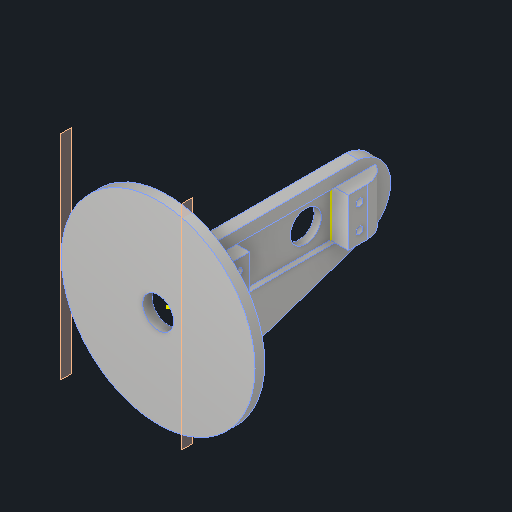
# Autodesk Inventor part: wrist
Saved by Autodesk Inventor 2023.4 (Build 274418000, 418)
## iProperties
Created: 2020-06-03
Part Number: wrist
Material: Aluminum 6061
Document SubType Name: Modeling
Designer: lenovo
Density: 2.7 g/cm^3
Appearance: Aluminum - Flat
Author: lenovo
Autodesk Inventor part; units mm, degrees
ref_plane "XZ Plane" through (0, 0, 0) normal (0, 1, 0) x (-1, 0, 0)
ref_plane "XY Plane" through (0, 0, 0) normal (0, 0, 1) x (1, 0, 0)
sketch "Sketch1" plane through (0, 0, 0) normal (0, 0, 1) x (1, 0, 0)
  circle A0 centre (0, 0) radius 40
  dimension "d0" = 80
  constraints: 1 centre point, 1 coincident
  measures "d0" diameter of A0
extrude "Extrusion1" add sketch "Sketch1" along normal blind 4
ref_plane "Work Plane2" through (10, 0, 0) normal (1, 0, 0) x (0, 1, 0)
ref_plane "Work Plane1" through (-40, 0, 0) normal (1, 0, 0) x (0, 1, 0)
sketch "Sketch2" plane through (10, 0, 0) normal (1, 0, 0) x (0, 1, 0)
  line L0 (-21.6965, 0) -> (-21.6965, -5)
  line L1 (-21.6965, -5) -> (28.3035, -5)
  line L2 (28.3035, -5) -> (28.3035, 0)
  circle A0 centre (13.3035, -44.0044) radius 10
  line L3 (-21.6965, -5) -> (0, -41.2491)
  line L4 (28.3035, -5) -> (23.2249, -45.256)
  line L5 (-21.6965, 0) -> (28.3035, 0)
  line L6 (28.3035, -5) -> (28.3035, -63.6411)
  arc A1 (0, -69.0405) -> (28.3035, -60.1475) centre (13.3035, -61.8943) ccw
  arc A2 (4.8652, -49.3705) -> (4.8622, -49.3725) centre (13.3035, -61.8943) ccw
  line L7 (0, -69.0405) -> (-21.6965, -5)
  point P0 (0, 0)
  point P1 (11.1199, -34.2457)
  point P2 (4.723, -49.1401)
  dimension "d4" = 5
  dimension "d5" = 50
  dimension "d6" = 20
  dimension "d8" = 15
  constraints: 16 end point, 9 point on circle, 3 centre point, 2 perpendicular, 2 point on line, 2 tangent, 2 vertical, 1 horizontal
  measures "d4" distance of L0.start L0.end
  measures "d5" distance of L0.end L1.end
  measures "d6" diameter of A0
  measures "d8" distance from line of L2 A0.centre
extrude "Extrusion4" add sketch "Sketch2" along normal blind 5 contours L5 L2 L1 L0 | L1 L6 A1 L7 | A0
sketch "Sketch3" plane through (10, 0, 0) normal (-1, 0, 0) x (0, 0, 1)
  arc A0 (-45.256, 23.2249) -> (-49.1401, 4.723) centre (-44.0044, 13.3035) ccw projected
  circle A1 centre (-44.0044, 13.3035) radius 6.4
  point P0 (0, 0)
  dimension "d15" = 12.8
  constraints: 1 centre point, 1 coincident
  measures "d15" diameter of A1
extrude "Extrusion5" cut sketch "Sketch3" against normal through all
sketch "Sketch6" plane through (15, 0, 0) normal (1, 0, 0) x (0, 0, -1)
  point P0 (0, 0)
sketch "Sketch7" plane through (15, 0, 0) normal (1, 0, 0) x (0, 0, -1)
  line L0 (13.4044, 3.4035) -> (54.0044, 3.4035)
  line L1 (54.0044, 3.4035) -> (54.0044, 23.2035)
  line L2 (54.0044, 23.2035) -> (13.4044, 23.2035)
  line L3 (13.4044, 23.2035) -> (13.4044, 3.4035)
  line L4 (13.4044, 3.4035) -> (54.0044, 23.2035) construction
  line L5 (54.0044, 3.4035) -> (13.4044, 23.2035) construction
  circle A0 centre (44.0044, 13.3035) radius 6.4 projected
  point P0 (0, 0)
  point P1 (33.7044, 13.3035)
  dimension "d24" = 40.6
  dimension "d25" = 19.8
  dimension "d35" = 9.9
  dimension "d36" = 10
  constraints: 12 end point, 2 midpoint, 2 parallel, 1 horizontal, 1 perpendicular
  measures "d24" distance of L2.end L1.end
  measures "d25" distance of L0.end L1.end
  measures "d35" distance from line of L2 A0.centre
  measures "d36" distance from line of L1 A0.centre
extrude "Extrusion8" cut sketch "Sketch7" against normal blind 2 contours L3 L2 L1 L0 | A0
sketch "Sketch8" plane through (15, 0, 0) normal (1, 0, 0) x (0, 0, -1)
  line L0 (54.0044, 23.2035) -> (54.0044, 3.4035) projected
  line L1 (54.0044, 23.2035) -> (64.0044, 23.2035)
  line L2 (64.0044, 23.2035) -> (64.0044, 3.4035)
  line L3 (64.0044, 3.4035) -> (54.0044, 3.4035)
  line L4 (54.0044, 3.4035) -> (54.0044, 23.2035)
  point P0 (0, 0)
  dimension "d28" = 10
  dimension "d29" = 19.8
  constraints: 8 end point, 2 parallel, 1 horizontal, 1 perpendicular
  measures "d28" distance of L2.end L3.end
  measures "d29" distance of L1.end L2.end
extrude "Extrusion9" add sketch "Sketch8" along normal blind 5.5
sketch "Sketch9" plane through (15, 0, 0) normal (1, 0, 0) x (0, 0, -1)
  line L0 (64.0044, 23.2035) -> (64.0044, 3.4035) projected
  line L1 (64.0044, 23.2035) -> (70.7533, 23.2035)
  line L2 (70.7533, 23.2035) -> (70.7533, 3.4035)
  line L3 (70.7533, 3.4035) -> (64.0044, 3.4035)
  line L4 (64.0044, 3.4035) -> (64.0044, 23.2035)
  point P0 (0, 0)
  constraints: 8 end point, 2 parallel, 1 horizontal, 1 perpendicular
extrude "Extrusion10" add sketch "Sketch9" along normal blind 5.5
fillet "Fillet1" radius 10 1 edges at (20.5, 13.3035, -70.7533)
sketch "Sketch10" plane through (15, 0, 0) normal (1, 0, 0) x (0, 0, -1)
  line L0 (13.4044, 3.4035) -> (13.4044, 23.2035)
  line L1 (13.4044, 3.4035) -> (13.4044, 23.2035) projected
  line L2 (13.4044, 23.2035) -> (0.0004, 23.2035)
  line L3 (0.0004, 23.2035) -> (0.0004, 3.4035)
  line L4 (0.0004, 3.4035) -> (13.4044, 3.4035)
  line L5 (13.4044, 3.4035) -> (13.4044, 23.2035)
  point P0 (0, 0)
  dimension "d38" = 13.404
  constraints: 10 end point, 2 parallel, 1 horizontal, 1 perpendicular
  measures "d38" distance of L4.end L3.end
extrude "Extrusion11" add sketch "Sketch10" along normal blind 5.5
sketch "Sketch11" plane through (20.5, 0, 0) normal (1, 0, 0) x (0, 0, -1)
  line L0 (0.0004, 23.2035) -> (13.4044, 23.2035) projected
  line L1 (13.4044, 23.2035) -> (8.8144, 23.2035)
  line L2 (13.4044, 18.3035) -> (13.4044, 23.2035)
  circle A0 centre (8.8144, 18.3035) radius 1.475
  line L3 (13.4044, 3.4035) -> (13.4044, 23.2035) projected
  line L4 (13.4044, 13.3035) -> (0.0004, 13.3035)
  line L5 (0.0004, 3.4035) -> (0.0004, 23.2035) projected
  circle A1 centre (8.8144, 8.3035) radius 1.475
  point P0 (0, 0)
  dimension "d43" = 2.95
  dimension "d44" = 2.95
  constraints: 6 end point, 2 centre point, 2 midpoint, 1 coincident, 1 horizontal
  measures "d43" diameter of A0
  measures "d44" diameter of A1
extrude "Extrusion12" cut sketch "Sketch11" against normal blind 10 contours A0 | A1
sketch "Sketch12" plane through (20.5, 0, 0) normal (1, 0, 0) x (0, 0, -1)
  point P0 (0, 0)
sketch "Sketch13" plane through (10.5, 18.3035, -8.8144) normal (1, 0, 0) x (0, 0, -1)
  point P0 (-8.8144, -18.3035)
sketch "Sketch14" plane through (13, 0, 0) normal (1, 0, 0) x (0, 0, -1)
  circle A0 centre (8.8144, 18.3035) radius 1.475 projected
  line L0 (61.7531, 18.3035) -> (54.0044, 18.3035)
  line L1 (54.0044, 23.2035) -> (54.0044, 3.4035) projected
  point P0 (0, 0)
  constraints: 2 end point, 1 point on line
sketch "Sketch15" plane through (20.5, 0, 0) normal (1, 0, 0) x (0, 0, -1)
  circle A0 centre (8.8144, 18.3035) radius 1.475 projected
  line L0 (61.823, 23.2035) -> (61.823, 3.4035) projected
  circle A1 centre (8.8144, 8.3035) radius 1.475 projected
  line L1 (54.0044, 23.2035) -> (54.0044, 3.4035) projected
  circle A2 centre (58.5944, 18.3035) radius 1.475
  circle A3 centre (58.5944, 8.3035) radius 1.475
  point P0 (0, 0)
  dimension "d49" = 2.95
  dimension "d50" = 2.95
  constraints: 2 centre point
  measures "d49" diameter of A2
  measures "d50" diameter of A3
extrude "Extrusion13" cut sketch "Sketch15" against normal blind 10 contours A2 | A3
thread "Thread1" size "M3x0.5" class "6H" standard "ANSI Metric M Profile" full length
thread "Thread2" size "M3x0.5" class "6H" standard "ANSI Metric M Profile" full length
thread "Thread3" size "M3x0.5" class "6H" standard "ANSI Metric M Profile" full length
thread "Thread4" size "M3x0.5" class "6H" standard "ANSI Metric M Profile" full length
sketch "Sketch16" plane through (13, 0, 0) normal (1, 0, 0) x (0, 0, -1)
  point P0 (0, 0)
sketch "Sketch17" plane through (13, 0, 0) normal (1, 0, 0) x (0, 0, -1)
  point P0 (0, 0)
sketch "Sketch18" plane through (20.5, 0, 0) normal (1, 0, 0) x (0, 0, -1)
  point P0 (0, 0)
sketch "Sketch19" plane through (13, 0, 0) normal (1, 0, 0) x (0, 0, -1)
  point P0 (0, 0)
sketch "Sketch20" plane through (13, 0, 0) normal (1, 0, 0) x (0, 0, -1)
  point P0 (0, 0)
sketch "Sketch21" plane through (0, 0, 0) normal (0, 0, -1) x (-1, 0, 0)
  circle A0 centre (0, 0) radius 6.4
  dimension "d61" = 12.8
  constraints: 1 centre point, 1 coincident
  measures "d61" diameter of A0
extrude "Extrusion14" cut sketch "Sketch21" against normal blind 10
sketch "Sketch22" plane through (13, 0, 0) normal (1, 0, 0) x (0, 0, -1)
  point P0 (0, 0)
sketch "Sketch23" plane through (0, 0, 0) normal (0, 0, -1) x (-1, 0, 0)
  point P0 (0, 0)
sketch "Sketch24" plane through (0, 0, 0) normal (0, 0, -1) x (-1, 0, 0)
  point P0 (0, 0)
sketch "Sketch25" plane through (0, 0, 0) normal (0, 0, -1) x (-1, 0, 0)
  point P0 (0, 0)
body "Solid1"
